Autodesk Inventor part; units mm, degrees
(part 2 of 2)
sketch "Эскиз19" plane through (-553.2789, -264.3002, 1.4222) normal (0, -1, 0) x (1, 0, 0)
  line L0 (41.9631, 0) -> (41.9631, -7) projected
  line L1 (41.9631, 0) -> (35.9631, 0) projected
  line L2 (35.9631, -7) -> (35.9631, 0) projected
  line L3 (41.9631, -7) -> (35.9631, -7) projected
  circle A0 centre (38.9631, 8) radius 1.75 projected
  line L4 (41.9631, 23) -> (41.9631, 16) projected
  line L5 (41.9631, 23) -> (35.9631, 23) projected
  line L6 (35.9631, 16) -> (35.9631, 23) projected
  line L7 (41.9631, 16) -> (35.9631, 16) projected
  line L8 (490.3726, 65.8677) -> (-34.6354, 65.8677) projected
  line L9 (35.9631, 109) -> (35.9631, 116) projected
  line L10 (41.9631, 109) -> (35.9631, 109) projected
  line L11 (41.9631, 116) -> (41.9631, 109) projected
  line L12 (35.9631, 116) -> (41.9631, 116) projected
  circle A1 centre (38.9631, 124) radius 1.75 projected
  line L13 (41.9631, 132) -> (35.9631, 132) projected
  line L14 (35.9631, 132) -> (35.9631, 139) projected
  line L15 (35.9631, 139) -> (41.9631, 139) projected
  line L16 (41.9631, 139) -> (41.9631, 132) projected
  line L17 (135.0844, 0) -> (141.0844, 0) projected
  line L18 (135.0844, -7) -> (135.0844, 0) projected
  line L19 (135.3247, -7) -> (136.6297, -7) projected
  line L20 (141.0844, -7) -> (135.0844, -7) projected
  line L21 (141.0844, 0) -> (141.0844, -7) projected
  line L22 (135.0844, 16) -> (135.0844, 23) projected
  line L23 (141.0844, 16) -> (135.0844, 16) projected
  line L24 (141.0844, 23) -> (141.0844, 16) projected
  line L25 (135.0844, 23) -> (141.0844, 23) projected
  circle A2 centre (138.0844, 8) radius 1.75 projected
  line L26 (135.0844, 109) -> (135.0844, 116) projected
  line L27 (135.0844, 116) -> (141.0844, 116) projected
  line L28 (141.0844, 109) -> (135.0844, 109) projected
  line L29 (141.0844, 116) -> (141.0844, 109) projected
  circle A3 centre (138.3833, 122.178) radius 0.9 projected
  circle A4 centre (138.0844, 124) radius 1.75 projected
  line L30 (188.2269, 146.409) -> (188.2269, 95.659) projected
  line L31 (188.2269, 95.659) -> (164.2269, 95.659) projected
  line L32 (164.2269, 95.659) -> (164.2269, 146.409) projected
  line L33 (164.2269, 146.409) -> (188.2269, 146.409) projected
  line L34 (141.0844, 23) -> (141.0844, 16) projected
  line L35 (141.0844, 16) -> (135.0844, 16) projected
  line L36 (135.0844, 16) -> (135.0844, 23) projected
  line L37 (135.0844, 23) -> (141.0844, 23) projected
  line L38 (35.9631, 132) -> (35.9631, 139) projected
  line L39 (35.9631, 139) -> (41.9631, 139) projected
  line L40 (41.9631, 139) -> (41.9631, 132) projected
  line L41 (41.9631, 132) -> (35.9631, 132) projected
  circle A5 centre (38.9631, 8) radius 1.75 projected
  line L42 (41.9631, -7) -> (35.9631, -7) projected
  line L43 (35.9631, -7) -> (35.9631, 0) projected
  line L44 (35.9631, 0) -> (41.9631, 0) projected
  line L45 (41.9631, 0) -> (41.9631, -7) projected
  line L46 (141.0844, 139) -> (141.0844, 132) projected
  line L47 (141.0844, 132) -> (135.0844, 132) projected
  line L48 (135.0844, 132) -> (135.0844, 139) projected
  line L49 (135.0844, 139) -> (141.0844, 139) projected
  circle A6 centre (138.0844, 8) radius 1.75 projected
  line L50 (141.0844, 116) -> (141.0844, 109) projected
  line L51 (141.0844, 109) -> (135.0844, 109) projected
  line L52 (135.0844, 109) -> (135.0844, 116) projected
  line L53 (135.0844, 116) -> (141.0844, 116) projected
  circle A7 centre (38.9631, 124) radius 1.75 projected
  line L54 (41.9631, 16) -> (35.9631, 16) projected
  line L55 (35.9631, 16) -> (35.9631, 23) projected
  line L56 (35.9631, 23) -> (41.9631, 23) projected
  line L57 (41.9631, 23) -> (41.9631, 16) projected
  line L58 (35.9631, 109) -> (35.9631, 116) projected
  line L59 (35.9631, 116) -> (41.9631, 116) projected
  line L60 (41.9631, 116) -> (41.9631, 109) projected
  line L61 (41.9631, 109) -> (35.9631, 109) projected
  circle A8 centre (138.0844, 124) radius 1.75 projected
  line L62 (141.0844, 0) -> (141.0844, -7) projected
  line L63 (141.0844, -7) -> (135.0844, -7) projected
  line L64 (135.0844, -7) -> (135.0844, 0) projected
  line L65 (135.0844, 0) -> (141.0844, 0) projected
  circle A9 centre (130.9111, -16.5023) radius 1.2859 projected
  circle A10 centre (209.5461, 19.0176) radius 1.3005 projected
  circle A11 centre (130.9552, 19.0345) radius 1.2516 projected
  circle A12 centre (209.4904, -16.5085) radius 1.3414 projected
  circle A13 centre (194.5237, 85.5) radius 1.6 projected
  spline S0 degree 3 poles (38.7737, 66.1) (38.7737, 66.2887) (38.8115, 66.4898) (38.9647, 66.8592) (39.0801, 67.0277) (39.3461, 67.2936) (39.5145, 67.409) (39.884, 67.5622) (40.085, 67.6) (40.4625, 67.6) (40.6635, 67.5622) (41.033, 67.409) (41.2014, 67.2936) (41.4674, 67.0277) (41.5828, 66.8592) (41.7359, 66.4898) (41.7737, 66.2887) (41.7737, 65.9113) (41.7359, 65.7102) (41.5828, 65.3408) (41.4674, 65.1723) (41.2014, 64.9064) (41.033, 64.791) (40.6635, 64.6378) (40.4625, 64.6) (40.085, 64.6) (39.884, 64.6378) (39.5145, 64.791) (39.3461, 64.9064) (39.0801, 65.1723) (38.9647, 65.3408) (38.8115, 65.7102) (38.7737, 65.9113) (38.7737, 66.1) knots 0 0 0 0 0.056617 0.056617 0.113235 0.113235 0.169851 0.169851 0.226467 0.226467 0.283083 0.283083 0.339699 0.339699 0.396316 0.396316 0.452934 0.452934 0.509551 0.509551 0.566168 0.566168 0.622784 0.622784 0.6794 0.6794 0.736016 0.736016 0.792632 0.792632 0.84925 0.84925 0.905867 0.905867 0.905867 0.905867 projected
  spline S1 degree 3 poles (-19.7263, 65.9) (-19.7263, 65.7113) (-19.7641, 65.5102) (-19.9172, 65.1408) (-20.0326, 64.9723) (-20.2986, 64.7064) (-20.467, 64.591) (-20.8365, 64.4378) (-21.0375, 64.4) (-21.415, 64.4) (-21.616, 64.4378) (-21.9855, 64.591) (-22.1539, 64.7064) (-22.4199, 64.9723) (-22.5353, 65.1408) (-22.6885, 65.5102) (-22.7263, 65.7113) (-22.7263, 66.0887) (-22.6885, 66.2898) (-22.5353, 66.6592) (-22.4199, 66.8277) (-22.1539, 67.0936) (-21.9855, 67.209) (-21.616, 67.3622) (-21.415, 67.4) (-21.0375, 67.4) (-20.8365, 67.3622) (-20.467, 67.209) (-20.2986, 67.0936) (-20.0326, 66.8277) (-19.9172, 66.6592) (-19.7641, 66.2898) (-19.7263, 66.0887) (-19.7263, 65.9) knots 0 0 0 0 0.056617 0.056617 0.113235 0.113235 0.169851 0.169851 0.226467 0.226467 0.283083 0.283083 0.339699 0.339699 0.396316 0.396316 0.452934 0.452934 0.509551 0.509551 0.566168 0.566168 0.622784 0.622784 0.6794 0.6794 0.736016 0.736016 0.792632 0.792632 0.84925 0.84925 0.905867 0.905867 0.905867 0.905867 projected
  circle A14 centre (132.5237, 149.5) radius 1.6 projected
  circle A15 centre (132.5237, 37.5) radius 1.6 projected
  circle A16 centre (132.5237, 85.5) radius 1.6 projected
  spline S2 degree 3 poles (21.2737, 65.9) (21.2737, 65.7113) (21.2359, 65.5102) (21.0828, 65.1408) (20.9674, 64.9723) (20.7014, 64.7064) (20.533, 64.591) (20.1635, 64.4378) (19.9625, 64.4) (19.585, 64.4) (19.384, 64.4378) (19.0145, 64.591) (18.8461, 64.7064) (18.5801, 64.9723) (18.4647, 65.1408) (18.3115, 65.5102) (18.2737, 65.7113) (18.2737, 66.0887) (18.3115, 66.2898) (18.4647, 66.6592) (18.5801, 66.8277) (18.8461, 67.0936) (19.0145, 67.209) (19.384, 67.3622) (19.585, 67.4) (19.9625, 67.4) (20.1635, 67.3622) (20.533, 67.209) (20.7014, 67.0936) (20.9674, 66.8277) (21.0828, 66.6592) (21.2359, 66.2898) (21.2737, 66.0887) (21.2737, 65.9) knots 0 0 0 0 0.056617 0.056617 0.113235 0.113235 0.169851 0.169851 0.226467 0.226467 0.283083 0.283083 0.339699 0.339699 0.396316 0.396316 0.452934 0.452934 0.509551 0.509551 0.566168 0.566168 0.622784 0.622784 0.6794 0.6794 0.736016 0.736016 0.792632 0.792632 0.84925 0.84925 0.905867 0.905867 0.905867 0.905867 projected
  spline S3 degree 3 poles (-2.2263, 66.1) (-2.2263, 66.2887) (-2.1885, 66.4898) (-2.0353, 66.8592) (-1.9199, 67.0277) (-1.6539, 67.2936) (-1.4855, 67.409) (-1.116, 67.5622) (-0.915, 67.6) (-0.5375, 67.6) (-0.3365, 67.5622) (0.033, 67.409) (0.2014, 67.2936) (0.4674, 67.0277) (0.5828, 66.8592) (0.7359, 66.4898) (0.7737, 66.2887) (0.7737, 65.9113) (0.7359, 65.7102) (0.5828, 65.3408) (0.4674, 65.1723) (0.2014, 64.9064) (0.033, 64.791) (-0.3365, 64.6378) (-0.5375, 64.6) (-0.915, 64.6) (-1.116, 64.6378) (-1.4855, 64.791) (-1.6539, 64.9064) (-1.9199, 65.1723) (-2.0353, 65.3408) (-2.1885, 65.7102) (-2.2263, 65.9113) (-2.2263, 66.1) knots 0 0 0 0 0.056617 0.056617 0.113235 0.113235 0.169851 0.169851 0.226467 0.226467 0.283083 0.283083 0.339699 0.339699 0.396316 0.396316 0.452934 0.452934 0.509551 0.509551 0.566168 0.566168 0.622784 0.622784 0.6794 0.6794 0.736016 0.736016 0.792632 0.792632 0.84925 0.84925 0.905867 0.905867 0.905867 0.905867 projected
  circle A17 centre (194.5237, 149.5) radius 1.6 projected
  circle A18 centre (194.5237, 37.5) radius 1.6 projected
  line L66 (18.5237, 115.5) -> (18.5237, 105.5) projected
  line L67 (18.5237, 105.5) -> (-26.4763, 105.5) projected
  line L68 (-26.4763, 105.5) -> (-26.4763, 115.5) projected
  line L69 (-26.4763, 115.5) -> (18.5237, 115.5) projected
  line L70 (18.5237, 26.5) -> (18.5237, 16.5) projected
  line L71 (18.5237, 16.5) -> (-26.4763, 16.5) projected
  line L72 (-26.4763, 16.5) -> (-26.4763, 26.5) projected
  line L73 (-26.4763, 26.5) -> (18.5237, 26.5) projected
  circle A19 centre (0, -28.25) radius 1.75 projected
  circle A20 centre (0, 160.25) radius 1.75 projected
  circle A21 centre (195.0475, 160.25) radius 1.75 projected
  circle A22 centre (195.0475, -28.25) radius 1.75 projected
  circle A23 centre (177.0475, 160.25) radius 1.75 projected
  circle A24 centre (-18, 160.25) radius 1.75 projected
  circle A25 centre (-18, -28.25) radius 1.75 projected
  circle A26 centre (18, 160.25) radius 1.75 projected
  circle A27 centre (159.0475, -28.25) radius 1.75 projected
  circle A28 centre (177.0475, -28.25) radius 1.75 projected
  circle A29 centre (159.0475, 160.25) radius 1.75 projected
  circle A30 centre (18, -28.25) radius 1.75 projected
  circle A31 centre (53.5237, 156) radius 5 projected
  circle A32 centre (53.5237, -24) radius 5 projected
  line L74 (66.0237, 157.5) -> (111.0237, 157.5) projected
  line L75 (111.0237, 157.5) -> (111.0237, -25.5) projected
  line L76 (111.0237, -25.5) -> (66.0237, -25.5) projected
  line L77 (66.0237, -25.5) -> (66.0237, 157.5) projected
  line L78 (204.5237, 93.5765) -> (216.5237, 93.5765) projected
  line L79 (216.5237, 93.5765) -> (216.5237, 38.5765) projected
  line L80 (216.5237, 38.5765) -> (204.5237, 38.5765) projected
  line L81 (204.5237, 38.5765) -> (204.5237, 93.5765) projected
  circle A33 centre (-43.4763, 18.5) radius 1.75 projected
  circle A34 centre (-43.4763, 55.625) radius 1.75 projected
  circle A35 centre (-43.4763, 113.5) radius 1.75 projected
  circle A36 centre (-43.4763, 76.375) radius 1.75 projected
  arc A37 (-38.4763, 163.5) -> (-46.4763, 155.5) centre (-38.4763, 155.5) ccw projected
  line L82 (-46.4763, 155.5) -> (-46.4763, 143.5) projected
  line L83 (-46.4763, 143.5) -> (-40.4763, 143.5) projected
  line L84 (-40.4763, 143.5) -> (-40.4763, 123.5) projected
  line L85 (-40.4763, 123.5) -> (-46.4763, 123.5) projected
  line L86 (-46.4763, 123.5) -> (-46.4763, 103.5) projected
  line L87 (-46.4763, 103.5) -> (-40.4763, 103.5) projected
  line L88 (-40.4763, 103.5) -> (-40.4763, 83.5) projected
  line L89 (-40.4763, 83.5) -> (-46.4763, 83.5) projected
  line L90 (-46.4763, 83.5) -> (-46.4763, 48.5) projected
  line L91 (-46.4763, 48.5) -> (-40.4763, 48.5) projected
  line L92 (-40.4763, 48.5) -> (-40.4763, 28.5) projected
  line L93 (-40.4763, 28.5) -> (-46.4763, 28.5) projected
  line L94 (-46.4763, 28.5) -> (-46.4763, 8.5) projected
  line L95 (-46.4763, 8.5) -> (-40.4763, 8.5) projected
  line L96 (-40.4763, 8.5) -> (-40.4763, -11.5) projected
  line L97 (-40.4763, -11.5) -> (-46.4763, -11.5) projected
  line L98 (-46.4763, -11.5) -> (-46.4763, -23.5) projected
  arc A38 (-46.4763, -23.5) -> (-38.4763, -31.5) centre (-38.4763, -23.5) ccw projected
  line L99 (-38.4763, -31.5) -> (26, -31.5) projected
  arc A39 (30, -35.5) -> (26, -31.5) centre (22.7085, -38.7915) ccw projected
  line L100 (30, -35.5) -> (30, -39) projected
  arc A40 (30, -39) -> (38, -47) centre (38, -39) ccw projected
  line L101 (38, -47) -> (138.803, -47) projected
  arc A41 (138.803, -47) -> (146.803, -39) centre (138.803, -39) ccw projected
  line L102 (146.803, -39) -> (146.803, -35.5) projected
  arc A42 (150.803, -31.5) -> (146.803, -35.5) centre (154.0945, -38.7915) ccw projected
  line L103 (150.803, -31.5) -> (215.5237, -31.5) projected
  arc A43 (215.5237, -31.5) -> (223.5237, -23.5) centre (215.5237, -23.5) ccw projected
  line L104 (223.5237, -23.5) -> (223.5237, 155.5) projected
  arc A44 (223.5237, 155.5) -> (215.5237, 163.5) centre (215.5237, 155.5) ccw projected
  line L105 (215.5237, 163.5) -> (150.803, 163.5) projected
  arc A45 (146.803, 167.7701) -> (150.803, 163.5) centre (154.2371, 170.7254) ccw projected
  line L106 (146.803, 167.7701) -> (146.803, 171.2701) projected
  arc A46 (146.803, 171.2701) -> (138.803, 179.2701) centre (138.803, 171.2701) ccw projected
  line L107 (138.803, 179.2701) -> (38.2701, 179.2701) projected
  arc A47 (38.2701, 179.2701) -> (30.2701, 171.2701) centre (38.2701, 171.2701) ccw projected
  line L108 (30.2701, 171.2701) -> (30.2701, 167.7701) projected
  arc A48 (26, 163.5) -> (30.2701, 167.7701) centre (22.8966, 170.8735) ccw projected
  line L109 (26, 163.5) -> (-38.4763, 163.5) projected
  circle A49 centre (111.0237, -35.5) radius 2 projected
  circle A50 centre (88.5237, -35.5) radius 2 projected
  circle A51 centre (66.0237, -35.5) radius 2 projected
  circle A52 centre (111.0237, 167.5) radius 2 projected
  circle A53 centre (88.5237, 167.5) radius 2 projected
  circle A54 centre (66.0237, 167.5) radius 2 projected
  line L110 (130.5237, -7) -> (124.5237, -7)
  line L111 (124.5237, 0) -> (124.5237, -7)
  line L112 (130.5237, 0) -> (124.5237, 0)
  line L113 (130.5237, -7) -> (130.5237, 0)
  line L114 (130.5237, 16) -> (124.5237, 16)
  line L115 (124.5237, 23) -> (124.5237, 16)
  line L116 (130.5237, 23) -> (124.5237, 23)
  line L117 (130.5237, 16) -> (130.5237, 23)
  line L118 (130.5237, 139) -> (124.5237, 139)
  line L119 (130.5237, 132) -> (130.5237, 139)
  line L120 (130.5237, 132) -> (124.5237, 132)
  line L121 (124.5237, 139) -> (124.5237, 132)
  line L122 (130.5237, 116) -> (124.5237, 116)
  line L123 (130.5237, 109) -> (130.5237, 116)
  line L124 (130.5237, 109) -> (124.5237, 109)
  line L125 (124.5237, 116) -> (124.5237, 109)
  line L126 (130.5237, 122.25) -> (130.5237, 125.75)
  line L127 (124.5237, 125.75) -> (124.5237, 122.25)
  line L128 (130.5237, 6.25) -> (130.5237, 9.75)
  line L129 (124.5237, 9.75) -> (124.5237, 6.25)
  circle A55 centre (127.5237, 8) radius 1.75
  circle A56 centre (127.5237, 124) radius 1.75
  line L130 (111.4348, 132) -> (111.4348, 139)
  line L131 (111.4348, 109) -> (111.4348, 116)
  line L132 (117.4348, 109) -> (111.4348, 109)
  line L133 (117.4348, 116) -> (117.4348, 109)
  line L134 (117.4348, 116) -> (111.4348, 116)
  line L135 (117.4348, 132) -> (111.4348, 132)
  line L136 (117.4348, 139) -> (117.4348, 132)
  line L137 (117.4348, 139) -> (111.4348, 139)
  line L138 (111.4348, 122.25) -> (111.4348, 125.75)
  line L139 (117.4348, 125.75) -> (117.4348, 122.25)
  line L140 (117.4348, 122.25) -> (111.4348, 122.25)
  line L141 (117.4348, 125.75) -> (111.4348, 125.75)
  line L142 (111.4348, -0.2645) -> (111.4348, -7.2645)
  line L143 (111.4348, 22.7355) -> (111.4348, 15.7355)
  line L144 (117.4348, 22.7355) -> (111.4348, 22.7355)
  line L145 (117.4348, 15.7355) -> (117.4348, 22.7355)
  line L146 (117.4348, 15.7355) -> (111.4348, 15.7355)
  line L147 (117.4348, -0.2645) -> (111.4348, -0.2645)
  line L148 (117.4348, -7.2645) -> (117.4348, -0.2645)
  line L149 (117.4348, -7.2645) -> (111.4348, -7.2645)
  line L150 (111.4348, 9.4855) -> (111.4348, 5.9855)
  line L151 (117.4348, 5.9855) -> (117.4348, 9.4855)
  line L152 (117.4348, 9.4855) -> (111.4348, 9.4855)
  line L153 (117.4348, 5.9855) -> (111.4348, 5.9855)
  circle A57 centre (114.4348, 124) radius 1.75
  circle A58 centre (114.4348, 7.7355) radius 1.75
  point P0 (553.2789, -1.4222)
  point P1 (135.3367, -1.987)
  point P2 (38.7737, 66.1)
  point P3 (-19.7263, 65.9)
  point P4 (21.2737, 65.9)
  point P5 (-2.2263, 66.1)
  dimension "d23" = 8
  dimension "d24" = 8
  constraints: 88 end point, 18 vertical, 14 horizontal, 12 symmetric about line, 4 centre point, 42 other
extrude "Выдавливание18" cut sketch "Эскиз19" against normal blind 8 contours L0 L3 L2 L1 | A0 | L4 L7 L6 L5 | L9 L12 L11 L10 | A1 | L13 L14 L15 L16 | L130 L137 L136 L135 | L131 L134 L133 L132 | A57 | L147 L148 L149 L142 | L144 L145 L146 L143 | A58
sketch "Эскиз21" plane through (-553.2789, -260.3002, 1.4222) normal (0, 1, 0) x (1, 0, 0)
  circle A0 centre (20.333, -160.5) radius 2 projected
  circle A1 centre (20.333, -140.5) radius 2 projected
  circle A2 centre (-3.667, -160.5) radius 2 projected
  circle A3 centre (-3.667, -140.5) radius 2 projected
  circle A4 centre (20.333, 8.5) radius 2 projected
  circle A5 centre (20.333, 28.5) radius 2 projected
  circle A6 centre (-3.667, 8.5) radius 2 projected
  circle A7 centre (-3.667, 28.5) radius 2 projected
  point P0 (553.2789, 1.4222)
extrude "Выдавливание20" cut sketch "Эскиз21" against normal blind 10
chamfer "Фаска2" distance 1 angle 45 8 edges at (-558.9459, -260.3002, -27.0778) (-558.9459, -260.3002, -7.0778) (-534.9459, -260.3002, -27.0778) (-534.9459, -260.3002, -7.0778) (-534.9459, -260.3002, 141.9222) (-534.9459, -260.3002, 161.9222) (-558.9459, -260.3002, 161.9222) (-558.9459, -260.3002, 141.9222)
sketch "Эскиз26" plane through (-553.2789, -260.3002, 1.4222) normal (0, 1, 0) x (1, 0, 0)
  line L0 (30.2701, -167.7701) -> (146.803, -167.7701) projected
  line L1 (146.803, -167.7701) -> (30.2701, -167.7701)
  line L2 (30.2701, -167.7701) -> (30.2701, -168.2701)
  line L3 (32.2701, -170.2701) -> (144.803, -170.2701)
  line L4 (146.803, -168.2701) -> (146.803, -167.7701)
  arc A0 (146.803, 35.5) -> (150.803, 31.5) centre (154.0945, 38.7915) ccw projected
  line L5 (146.803, 35.5) -> (30, 35.5)
  line L6 (30, 35.5) -> (30, 36)
  line L7 (32, 38) -> (144.803, 38)
  line L8 (146.803, 36) -> (146.803, 35.5)
  arc A1 (32, 38) -> (30, 36) centre (32, 36) ccw
  arc A2 (146.803, 36) -> (144.803, 38) centre (144.803, 36) ccw
  arc A3 (144.803, -170.2701) -> (146.803, -168.2701) centre (144.803, -168.2701) ccw
  arc A4 (30.2701, -168.2701) -> (32.2701, -170.2701) centre (32.2701, -168.2701) ccw
  point P0 (553.2789, 1.4222)
  point P1 (50.5237, -167.7701)
  point P2 (146.803, -170.2701)
  point P3 (30, 38)
  point P4 (50.5237, -167.7701)
  dimension "d91" = 2.5
  dimension "d92" = 2.5
  dimension "d93" = 2
  constraints: 16 end point, 8 point on circle, 8 tangent, 4 centre point, 4 parallel, 4 point on line, 3 equal radius, 2 horizontal, 2 perpendicular
  measures "d91" distance of point (146.803, -170.27) L0.end
  measures "d92" distance of L5.end point (30, 38)
  measures "d93" radius of A1
extrude "Выдавливание25" add sketch "Эскиз26" against normal blind 4
sketch "Эскиз30" plane through (-553.2789, -260.3002, 1.4222) normal (0, 1, 0) x (1, 0, 0)
  line L0 (150.803, -163.5) -> (168.5237, -163.5) projected
  line L1 (150.803, -163.5) -> (19.4725, -163.5)
  line L2 (19.4725, -163.5) -> (19.4725, -173.0882)
  line L3 (19.4725, -173.0882) -> (150.803, -173.0882)
  line L4 (150.803, -173.0882) -> (150.803, -163.5)
  line L5 (168.5237, 31.5) -> (150.803, 31.5) projected
  line L6 (150.803, 31.5) -> (13.1107, 31.5)
  line L7 (13.1107, 31.5) -> (13.1107, 42.898)
  line L8 (13.1107, 42.898) -> (150.803, 42.898)
  line L9 (150.803, 42.898) -> (150.803, 31.5)
  point P0 (553.2789, 1.4222)
  constraints: 16 end point, 4 parallel, 2 horizontal, 2 perpendicular
sketch "Эскиз32" plane through (-553.2789, -264.3002, 1.4222) normal (0, -1, 0) x (1, 0, 0)
  point P0 (553.2789, -1.4222)
  dimension "d23" = 8
  dimension "d24" = 8
sketch "Эскиз33" plane through (-553.2789, -264.3002, 1.4222) normal (0, -1, 0) x (1, 0, 0)
  arc A0 (150.803, -31.5) -> (146.803, -35.5) centre (154.0945, -38.7915) ccw projected
  line L0 (150.803, -31.5) -> (26, -31.5)
  line L1 (26, -31.5) -> (26, -41.6347)
  line L2 (26, -41.6347) -> (150.803, -41.6347)
  line L3 (150.803, -41.6347) -> (150.803, -31.5)
  line L4 (-38.4763, 163.5) -> (26, 163.5) projected
  line L5 (26, 163.5) -> (152.8141, 163.5)
  line L6 (152.8141, 163.5) -> (152.8141, 171.9546)
  line L7 (152.8141, 171.9546) -> (26, 171.9546)
  line L8 (26, 171.9546) -> (26, 163.5)
  point P0 (553.2789, -1.4222)
  dimension "d23" = 8
  dimension "d24" = 8
  constraints: 16 end point, 4 parallel, 2 horizontal, 2 perpendicular
extrude "Выдавливание30" cut sketch "Эскиз33" against normal blind 10
sketch "Эскиз34" plane through (-553.2789, -260.3002, 1.4222) normal (0, 1, 0) x (1, 0, 0)
  line L0 (142.5237, -12.8461) -> (164.5237, -12.8461)
  line L1 (164.5237, -12.8461) -> (164.5237, -18.8461)
  line L2 (164.5237, -18.8461) -> (142.5237, -18.8461)
  line L3 (142.5237, -12.8461) -> (142.5237, -18.8461)
  line L4 (164.5237, -12.8461) -> (142.5237, -12.8461)
  line L5 (142.5237, -12.8461) -> (142.5237, -18.8461)
  line L6 (142.5237, -18.8461) -> (164.5237, -18.8461)
  line L7 (164.5237, -18.8461) -> (164.5237, -12.8461)
  line L8 (176.5237, -155.5) -> (176.5237, 23.5) projected
  line L9 (176.5237, 23.5) -> (176.5237, -66)
  line L10 (176.5237, -66) -> (76.1362, -66)
  line L11 (142.5237, -119.1539) -> (164.5237, -119.1539)
  line L12 (164.5237, -119.1539) -> (164.5237, -113.1539)
  line L13 (164.5237, -113.1539) -> (142.5237, -113.1539)
  line L14 (142.5237, -119.1539) -> (142.5237, -113.1539)
  line L15 (164.5237, -119.1539) -> (142.5237, -119.1539)
  line L16 (142.5237, -119.1539) -> (142.5237, -113.1539)
  line L17 (142.5237, -113.1539) -> (164.5237, -113.1539)
  line L18 (164.5237, -113.1539) -> (164.5237, -119.1539)
  point P0 (553.2789, 1.4222)
  dimension "d111" = 89.5
  constraints: 36 end point, 6 symmetric about line, 4 horizontal, 2 parallel, 2 vertical, 1 midpoint, 1 perpendicular, 4 other
  measures "d111" distance of L8.end L9.end
extrude "Выдавливание31" cut sketch "Эскиз34" against normal blind 10
sketch "Эскиз35" plane through (-553.2789, -260.3002, 1.4222) normal (0, 1, 0) x (1, 0, 0)
  line L0 (138.2737, -12.8461) -> (138.2737, -18.8461)
  line L1 (133.2737, -12.8461) -> (133.2737, -18.8461)
  line L2 (139.7737, -12.8461) -> (139.7737, -18.8461)
  line L3 (134.7737, -18.8461) -> (134.7737, -12.8461)
  line L4 (134.7737, -12.8461) -> (138.2737, -12.8461)
  line L5 (138.2737, -12.8461) -> (138.2737, -18.8461)
  line L6 (138.2737, -18.8461) -> (134.7737, -18.8461)
  line L7 (134.7737, -18.8461) -> (134.7737, -12.8461)
  circle A0 centre (136.5237, -15.8461) radius 1.75
  line L8 (142.5237, -12.8461) -> (164.5237, -12.8461) projected
  line L9 (153.5237, -12.8461) -> (153.5237, -3.0623)
  line L10 (168.7737, -12.8461) -> (168.7737, -18.8461)
  line L11 (173.7737, -12.8461) -> (173.7737, -18.8461)
  line L12 (167.2737, -12.8461) -> (167.2737, -18.8461)
  line L13 (172.2737, -18.8461) -> (172.2737, -12.8461)
  line L14 (172.2737, -12.8461) -> (168.7737, -12.8461)
  line L15 (168.7737, -12.8461) -> (168.7737, -18.8461)
  line L16 (168.7737, -18.8461) -> (172.2737, -18.8461)
  line L17 (172.2737, -18.8461) -> (172.2737, -12.8461)
  circle A1 centre (170.5237, -15.8461) radius 1.75
  line L18 (176.5237, -155.5) -> (176.5237, 23.5) projected
  line L19 (176.5237, 23.5) -> (176.5237, -66)
  line L20 (176.5237, -66) -> (84.4337, -66)
  line L21 (138.2737, -119.1539) -> (138.2737, -113.1539)
  line L22 (133.2737, -119.1539) -> (133.2737, -113.1539)
  line L23 (139.7737, -119.1539) -> (139.7737, -113.1539)
  line L24 (134.7737, -113.1539) -> (134.7737, -119.1539)
  line L25 (134.7737, -119.1539) -> (138.2737, -119.1539)
  line L26 (138.2737, -119.1539) -> (138.2737, -113.1539)
  line L27 (138.2737, -113.1539) -> (134.7737, -113.1539)
  line L28 (134.7737, -113.1539) -> (134.7737, -119.1539)
  circle A2 centre (136.5237, -116.1539) radius 1.75
  line L29 (142.5237, -119.1539) -> (164.5237, -119.1539)
  line L30 (153.5237, -119.1539) -> (153.5237, -128.9377)
  line L31 (168.7737, -119.1539) -> (168.7737, -113.1539)
  line L32 (173.7737, -119.1539) -> (173.7737, -113.1539)
  line L33 (167.2737, -119.1539) -> (167.2737, -113.1539)
  line L34 (172.2737, -113.1539) -> (172.2737, -119.1539)
  line L35 (172.2737, -119.1539) -> (168.7737, -119.1539)
  line L36 (168.7737, -119.1539) -> (168.7737, -113.1539)
  line L37 (168.7737, -113.1539) -> (172.2737, -113.1539)
  line L38 (172.2737, -113.1539) -> (172.2737, -119.1539)
  circle A3 centre (170.5237, -116.1539) radius 1.75
  point P0 (553.2789, 1.4222)
  dimension "d112" = 89.5
  constraints: 74 end point, 37 symmetric about line, 5 vertical, 4 centre point, 2 horizontal, 2 midpoint, 2 parallel, 1 perpendicular, 11 other
  measures "d112" distance of L18.end L19.end
extrude "Выдавливание32" cut sketch "Эскиз35" against normal blind 10 contours A0 | A1 | A2 | A3
sketch "Эскиз36" plane through (-553.2789, -260.3002, 1.4222) normal (0, 1, 0) x (1, 0, 0)
  line L0 (146.5237, -81.3798) -> (146.5237, -50.6244)
  line L1 (140.9035, -45) -> (110.1481, -45)
  line L2 (103.5237, -88) -> (147.5237, -88)
  line L3 (147.5237, -88) -> (147.5237, -44)
  line L4 (147.5237, -44) -> (103.5237, -44)
  line L5 (103.5237, -44) -> (103.5237, -88)
  line L6 (103.5237, -88) -> (147.5237, -44) construction
  line L7 (147.5237, -88) -> (103.5237, -44) construction
  point P0 (553.2789, 1.4222)
  point P1 (125.5237, -66)
  dimension "d128" = 44
  dimension "d129" = 44
  dimension "d130" = 21
  dimension "d131" = 21
  constraints: 16 end point, 2 horizontal, 2 midpoint, 2 parallel, 1 perpendicular, 1 vertical, 4 other
  measures "d128" distance of L2.end L3.end
  measures "d129" distance of L3.end L4.end
  measures "d130" distance from line of L0 point (125.524, -66)
  measures "d131" distance from line of L1 point (125.524, -66)
extrude "Выдавливание33" cut sketch "Эскиз36" against normal blind 10
sketch "Эскиз37" plane through (-553.2789, -260.3002, 1.4222) normal (0, 1, 0) x (1, 0, 0)
  circle A0 centre (53.7682, 19) radius 2
  circle A1 centre (53.7682, -23.5) radius 2
  circle A2 centre (105.7682, 19) radius 2
  circle A3 centre (105.7682, -23.5) radius 2
  circle A4 centre (53.2792, -108.5) radius 2
  circle A5 centre (53.2792, -151) radius 2
  circle A6 centre (105.2792, -108.5) radius 2
  circle A7 centre (105.2792, -151) radius 2
  point P0 (553.2789, 1.4222)
  constraints: 8 centre point, 16 other
extrude "Выдавливание34" cut sketch "Эскиз37" against normal blind 10
sketch "Эскиз38" plane through (-553.2789, -260.3002, 1.4222) normal (0, 1, 0) x (1, 0, 0)
  ellipse E0 centre (-25.6894, -107) end of major axis (-25.6894, -109) minor radius 2
  ellipse E1 centre (-25.6894, -149.5) end of major axis (-25.6894, -151.5) minor radius 2
  ellipse E2 centre (26.3163, -149.5) end of major axis (26.3163, -147.5) minor radius 2
  ellipse E3 centre (26.3163, -107) end of major axis (26.3163, -105) minor radius 2
  point P0 (553.2789, 1.4222)
  constraints: 2 centre point, 10 other
extrude "Выдавливание35" cut sketch "Эскиз38" against normal blind 10
chamfer "Фаска3" distance 2 angle 45 16 edges at (-529.2789, -260.3002, -17.5778) (-581.2789, -260.3002, -17.5778) (-581.2789, -260.3002, 24.9222) (-529.2789, -260.3002, 24.9222) (-501.5106, -260.3002, -17.5778) (-501.5106, -260.3002, 24.9222) (-449.5106, -260.3002, -17.5778) (-449.5106, -260.3002, 24.9222) (-501.9996, -260.3002, 109.9222) (-501.9996, -260.3002, 152.4222) (-449.9996, -260.3002, 109.9222) (-449.9996, -260.3002, 152.4222) (-578.9683, -260.3002, 106.4222) (-578.9683, -260.3002, 148.9222) (-526.9626, -260.3002, 110.4222) (-526.9626, -260.3002, 152.9222)
sketch "Эскиз39" plane through (-553.2789, -260.3002, 1.4222) normal (0, 1, 0) x (1, 0, 0)
  point P0 (553.2789, 1.4222)
sketch "Эскиз40" plane through (-553.2789, -260.3002, 1.4222) normal (0, 1, 0) x (1, 0, 0)
  line L0 (103.5237, -38.6067) -> (147.5237, -38.6067)
  line L1 (147.5237, -38.6067) -> (147.5237, -30.7322)
  line L2 (147.5237, -30.7322) -> (103.5237, -30.7322)
  line L3 (103.5237, -30.7322) -> (103.5237, -38.6067)
  point P0 (553.2789, 1.4222)
  constraints: 8 end point, 2 parallel, 1 horizontal, 1 perpendicular
extrude "Выдавливание36" cut sketch "Эскиз40" against normal blind 10
sketch "Эскиз41" plane through (-553.2789, -260.3002, 1.4222) normal (0, 1, 0) x (1, 0, 0)
  line L0 (103.5237, -44) -> (147.5237, -44) projected
  line L1 (103.5237, -44) -> (93.5237, -44)
  line L2 (93.5237, -44) -> (93.5237, -88)
  line L3 (93.5237, -88) -> (103.5237, -88)
  line L4 (103.5237, -88) -> (103.5237, -44)
  point P0 (553.2789, 1.4222)
  dimension "d134" = 10
  constraints: 8 end point, 2 parallel, 1 horizontal, 1 perpendicular
  measures "d134" distance of L0.start L1.end
extrude "Выдавливание37" cut sketch "Эскиз41" against normal blind 10
